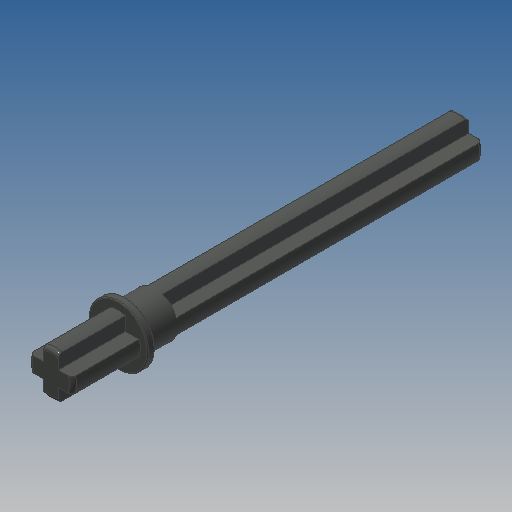
# Autodesk Inventor part: 32209-DkBluishGray
Saved by Autodesk Inventor 2022.2 (Build 262287000, 287)
## iProperties
Created: 2014-06-05
Part Number: 32209-DkBluishGray
Material: ABS Plastic
Document SubType Name: Modeling
Designer: D. Kohfeld
Density: 1.06 g/cm^3
Appearance: DkBluishGray
Mass: 0.616861 g
Surface Area: 8.48852 cm^2
Volume: 0.581945 cm^3
Description: Technic, Axle 5.5
Author: D. Kohfeld
Autodesk Inventor part; units mm, degrees
ref_plane "YZ Plane" through (0, 0, 0) normal (1, 0, 0) x (0, 1, 0)
ref_plane "XZ Plane" through (0, 0, 0) normal (0, 1, 0) x (-1, 0, 0)
sketch "Sketch1" plane through (0, 0, 0) normal (0, 0, 1) x (1, 0, 0)
  circle A0 centre (0, 0) radius 2.4 construction
  line L0 (-0.8, 2.2627) -> (-0.8, 0.8)
  line L1 (-0.8, 0.8) -> (-2.2627, 0.8)
  line L2 (-2.2627, -0.8) -> (-0.8, -0.8)
  line L3 (-0.8, -0.8) -> (-0.8, -2.2627)
  line L4 (0.8, -2.2627) -> (0.8, -0.8)
  line L5 (0.8, -0.8) -> (2.2627, -0.8)
  line L6 (2.2627, 0.8) -> (0.8, 0.8)
  line L7 (0.8, 0.8) -> (0.8, 2.2627)
  arc A1 (0.8, 2.2627) -> (-0.8, 2.2627) centre (0, 0) ccw
  arc A2 (-2.2627, 0.8) -> (-2.2627, -0.8) centre (0, 0) ccw
  arc A3 (-0.8, -2.2627) -> (0.8, -2.2627) centre (0, 0) ccw
  arc A4 (2.2627, -0.8) -> (2.2627, 0.8) centre (0, 0) ccw
  dimension "d0" = 4.8
  dimension "d1" = 1.6
  constraints: 16 end point, 8 point on circle, 7 equal length, 4 centre point, 4 perpendicular, 3 parallel, 1 coincident, 1 vertical, 14 other
  measures "d1" distance between parallel lines of L0 L7
extrude "Extrusion1" add sketch "Sketch1" along normal mid plane 44
ref_plane "Work Plane1" through (0, 0, 14) normal (0, 0, 1) x (1, 0, 0)
sketch "Sketch2" plane through (0, 0, 14) normal (0, 0, 1) x (1, 0, 0)
  circle A0 centre (0, 0) radius 3.2
  arc A1 (0.8, 2.2627) -> (-0.8, 2.2627) centre (0, 0) ccw projected
  circle A2 centre (0, 0) radius 2.4
  dimension "d8" = 6.4
  constraints: 2 coincident, 1 centre point, 3 other
  measures "d8" diameter of A0
extrude "Extrusion2" add sketch "Sketch2" along normal blind 0.8 contours A0 | A2 A1
extrude "Extrusion3" add sketch "Sketch2" against normal blind 3.2 contours A2 A1
fillet "Fillet1" radius 0.4 8 edges at (0, 2.4, 22) (-2.4, 0, 22) (0, -2.4, 22) (2.4, 0, 22) (2.4, 0, -22) (0, 2.4, -22) (-2.4, 0, -22) (0, -2.4, -22)
fillet "Fillet1" radius 0.1 2 edges at (-3.2, 0, 14.8) (-3.2, 0, 14)
equation "\"d0\" = kd"
equation "\"d1\" = axlet"
equation "\"d2\" = 5.5 * lu"
equation "\"d8\" = tsd"
equation "\"d9\" = tsl"
equation "\"d11\" = 0.5 * lu - tsl"
equation "\"d4\" = tf"
equation "\"d14\" = lf"
equation "\"kd\" = 4.8"
equation "\"axlet\" = 1.6"
equation "\"lu\" = 8"
equation "\"tsd\" = 6.4"
equation "\"tsl\" = 0.8"
equation "\"tf\" = 0.4"
equation "\"lf\" = 0.1"
body "Solid1"
